Cyclone  Mount Adapter (Autodesk Fusion 360 design; units mm, degrees)
Autodesk Fusion 360 part; units mm, degrees
sketch "Sketch1" plane through (0, 0, 0) normal (0, 0, 1) x (1, 0, 0)
  circle A0 centre (0, 0) radius 37.6
  circle A1 centre (0, 0) radius 45
  circle A2 centre (-45, 0) radius 2.5
  circle A3 centre (0.0008, 45) radius 2.5
  circle A4 centre (45, -0.0011) radius 2.5
  circle A5 centre (0.0001, -45) radius 2.5
  circle A6 centre (0, 0) radius 52.5
  dimension "d1" = 75.2
  dimension "d2" = 90
  dimension "d3" = 5
  dimension "d4" = 5
  dimension "d5" = 5
  dimension "d6" = 5
  dimension "d7" = 105
  constraint coincident A0.centre A1.centre
  constraint coincident A1 A2.centre
  constraint coincident A1 A3.centre
  constraint coincident A1 A4.centre
  constraint coincident A1 A5.centre
  constraint concentric A1 A6
  measures "d1" diameter of A0
  measures "d2" diameter of A1
  measures "d3" diameter of A2
  measures "d4" diameter of A3
  measures "d5" diameter of A4
  measures "d6" diameter of A5
  measures "d7" diameter of A6
extrude "Extrude1" add sketch "Sketch1" along normal blind 5 contours A1 A2 A3 A4 A5 | A6
